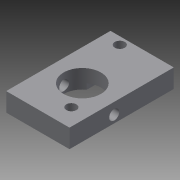
# Autodesk Inventor part: tapa0.2
Saved by Autodesk Inventor 2015 SP1 (Build 190203100, 203)
## iProperties
Created: 2015-06-09
Part Number: tapa0.2
Material: Generic
Document SubType Name: Modeling
Designer: pc
Density: 1 g/cm^3
Appearance: Default
Author: pc
Autodesk Inventor part; units mm, degrees
ref_plane "YZ Plane" through (0, 0, 0) normal (1, 0, 0) x (0, 1, 0)
ref_plane "XZ Plane" through (0, 0, 0) normal (0, 1, 0) x (-1, 0, 0)
ref_plane "XY Plane" through (0, 0, 0) normal (0, 0, 1) x (1, 0, 0)
sketch "Sketch2" plane through (0, 0, 0) normal (0, 0, 1) x (1, 0, 0)
  line L0 (-17, 28) -> (0, 28)
  line L1 (0, 28) -> (0, 17)
  line L2 (0, 7) -> (0, 0)
  line L3 (0, 0) -> (-17, 0)
  line L4 (-17, 0) -> (-17, 7)
  line L5 (-17, 28) -> (-17, 17)
  line L6 (-17, 17) -> (-17, 7)
  line L7 (0, 17) -> (0, 7)
  dimension "d0" = 17
  dimension "d1" = 28
  constraints: 16 end point, 3 perpendicular, 3 point on line, 1 coincident, 1 horizontal, 1 parallel, 1 vertical
  measures "d0" distance of L0.start L0.end
  measures "d1" distance between parallel lines of L0 L3
extrude "Extrusion1" add sketch "Sketch2" along normal blind 5
sketch "Sketch4" plane through (0, 0, 0) normal (0, 0, -1) x (-1, 0, 0)
  line L0 (17, 28) -> (0, 28) projected
  line L1 (0, 28) -> (0, 0) projected
  line L2 (0, 0) -> (17, 0) projected
  line L3 (17, 0) -> (17, 28) projected
  line L4 (0, 28) -> (17, 28) projected
  line L5 (11.5, 24) -> (11.5, 4)
  line L6 (11.5, 4) -> (5.5, 4)
  line L7 (5.5, 4) -> (5.5, 24)
  line L8 (5.5, 24) -> (11.5, 24)
  dimension "d15" = 6
  dimension "d17" = 5.5
  dimension "d30" = 20
  dimension "d31" = 4
  constraints: 8 end point, 1 parallel, 1 perpendicular
  measures "d15" distance of L5.end L6.end
  measures "d17" distance between parallel lines of L7 L1
  measures "d30" distance of L5.start L5.end
  measures "d31" distance between parallel lines of L2 L6
extrude "Extrusion3" cut sketch "Sketch4" against normal blind 1.5 contours L5 L6 L7 L8
sketch "Sketch5" plane through (0, 0, 5) normal (0, 0, 1) x (1, 0, 0)
  line L0 (0, 28) -> (-17, 28) projected
  line L1 (-17, 28) -> (-17, 0) projected
  line L2 (-17, 0) -> (0, 0) projected
  line L3 (0, 0) -> (0, 28) projected
  line L4 (-21, 17) -> (4, 7)
  line L5 (-21.4753, 7) -> (4, 17)
  circle A0 centre (-8.6177, 12.0471) radius 5
  dimension "d20" = 10
  dimension "d21" = 12.0471
  constraints: 4 end point, 2 point on line, 1 centre point
  measures "d20" diameter of A0
  measures "d21" distance from line of L2 A0.centre
extrude "Extrusion4" cut sketch "Sketch5" against normal through all contours A0 L4 L5 | L5 L4 A0 | L4 L5 A0 | A0 L5 L4
sketch "Sketch6" plane through (0, 0, 5) normal (0, 0, 1) x (1, 0, 0)
  circle A0 centre (-8.6177, 12.0471) radius 5 projected
  line L0 (0, 28) -> (-17, 28) projected
  line L1 (-17, 28) -> (-17, 0) projected
  line L2 (-17, 0) -> (0, 0) projected
  line L3 (0, 0) -> (0, 28) projected
  circle A1 centre (-12.5, 26) radius 1.35
  dimension "d24" = 2.7
  dimension "d25" = 4.5
  dimension "d26" = 2
  constraints: 1 centre point
  measures "d24" diameter of A1
  measures "d25" distance from line of A1.centre L1
  measures "d26" distance from line of L0 A1.centre
extrude "Extrusion5" cut sketch "Sketch6" against normal through all contours A1
sketch "Sketch7" plane through (0, 0, 5) normal (0, 0, 1) x (1, 0, 0)
  line L0 (0, 0) -> (0, 28) projected
  line L1 (-17, 0) -> (0, 0) projected
  circle A0 centre (-4.5, 5) radius 1.35
  point P0 (0, 7)
  dimension "d32" = 2.7
  dimension "d33" = 4.5
  dimension "d34" = 5
  constraints: 1 centre point
  measures "d32" diameter of A0
  measures "d33" distance from line of L0 A0.centre
  measures "d34" distance from line of L1 A0.centre
extrude "Extrusion6" cut sketch "Sketch7" against normal through all
sketch "Sketch8" plane through (0, 0, 0) normal (1, 0, 0) x (0, 0, -1)
  circle A0 centre (-2, 12) radius 1.35
  line L0 (-5, 0) -> (-5, 28) projected
  line L1 (0, 0) -> (-5, 0) projected
  point P0 (0, -7)
  dimension "d37" = 2.7
  dimension "d41" = 12
  constraints: 1 centre point
  measures "d37" diameter of A0
  measures "d41" distance from line of A0.centre L1
extrude "Extrusion8" cut sketch "Sketch8" against normal through all
body "Solid1"
